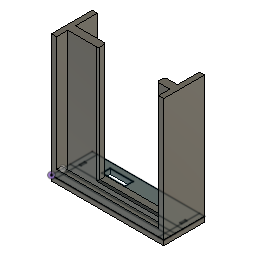
POWERDIAG_OBI_CASE_1 (Autodesk Fusion 360 design; units mm, degrees)
part number: 2026-08-31-19-42-01-999
Autodesk Fusion 360 part; units mm, degrees
sketch "Sketch1" plane through (0, 0, 0) normal (0, 0, 1) x (1, 0, 0)
  line L0 (0, 0) -> (44, 0)
  line L1 (44, 0) -> (44, 16)
  line L2 (44, 16) -> (0, 16)
  line L3 (0, 16) -> (0, 0)
  line L4 (0, 2.6) -> (44, 2.6)
  line L5 (2, 16) -> (2, 0)
  line L6 (42, 16) -> (42, 0)
  line L7 (0, 4.4) -> (44, 4.4)
  line L8 (0, 7.4) -> (44, 7.4)
  line L9 (9.2, 10.6) -> (18.2, 10.6)
  line L10 (18.2, 10.6) -> (18.2, 13.8)
  line L11 (18.2, 13.8) -> (9.2, 13.8)
  line L12 (9.2, 13.8) -> (9.2, 10.6)
  line L13 (2, 11) -> (2.6, 11)
  line L14 (2.6, 11) -> (2.6, 9)
  line L15 (2.6, 9) -> (2, 9)
  line L16 (2, 9) -> (2, 11)
  line L17 (42, 11) -> (41.4, 11)
  line L18 (41.4, 11) -> (41.4, 9)
  line L19 (41.4, 9) -> (42, 9)
  line L20 (42, 9) -> (42, 11)
  dimension "d2" = 16
  dimension "d3" = 2.6
  dimension "d4" = 2
  dimension "d5" = 2
  dimension "d7" = 1.8
  dimension "d8" = 3
  dimension "d9" = 3.2
  dimension "d10" = 3.2
  dimension "d11" = 9
  dimension "d12" = 7.2
  dimension "d13" = 40
  dimension "d22" = 2
  dimension "d23" = 0.6
  dimension "d24" = 1.6
  dimension "d25" = 1.6
  dimension "d26" = 0.6
  dimension "d27" = 2
  constraint horizontal L0
  constraint vertical L1
  constraint horizontal L2
  constraint vertical L3
  constraint coincident L0.start L3.end
  constraint coincident L3 L4.start
  constraint coincident L1 L4.end
  constraint perpendicular L1 L4
  constraint coincident L2 L5.start
  constraint coincident L0 L5.end
  constraint perpendicular L0 L5
  constraint coincident L2 L6.start
  constraint coincident L0 L6.end
  constraint perpendicular L0 L6
  constraint coincident L1 L7.end
  constraint perpendicular L1 L7
  constraint coincident L3 L8.start
  constraint perpendicular L6 L8
  constraint coincident L1 L8.end
  constraint horizontal L9
  constraint vertical L10
  constraint horizontal L11
  constraint vertical L12
  constraint horizontal L13
  constraint vertical L14
  constraint horizontal L15
  constraint vertical L16
  constraint coincident L5 L13.start
  constraint horizontal L17
  constraint vertical L18
  constraint horizontal L19
  constraint vertical L20
  constraint coincident L6 L17.start
  measures "d2" distance of L0.end L1.end
  measures "d3" distance of L0 L4
  measures "d4" distance of L3 L5
  measures "d5" distance of L1 L6
  measures "d7" distance of L4 L7
  measures "d8" distance of L7 L8
  measures "d9" distance of L8 L9
  measures "d10" distance of L9.start L11.end
  measures "d11" distance of L10 L12
  measures "d12" distance of L5 L12
  measures "d13" distance of L5 L6
  measures "d22" distance of L13.end L14.end
  measures "d23" distance of L5 L14
  measures "d24" distance of L8 L15
  measures "d25" distance of L8 L19
  measures "d26" distance of L18 L20
  measures "d27" distance of L17 L19
extrude "Extrude1" add sketch "Sketch1" against normal blind 2
extrude "Extrude2" add sketch "Sketch1" along normal blind 3 contours L0 L3 L4 L5 | L0 L4 L5 L6 | L3 L4 L5 L7 | L0 L1 L4 L6 | L3 L5 L7 L8 | L1 L4 L6 L7 | L5 L6 L7 L8 | L2 L3 L5 L8 L16 | L1 L6 L7 L8 | L1 L2 L6 L8 L20
sketch "Sketch2" plane through (0, 0, 3) normal (0, 0, 1) x (-1, 0, 0)
  line L0 (-2, -4.4) -> (-42, -4.4)
  line L1 (-42, -4.4) -> (-42, -2.6)
  line L2 (-42, -2.6) -> (-2, -2.6)
  line L3 (-2, -2.6) -> (-2, -4.4)
  line L4 (0, -16) -> (0, 0)
  line L5 (0, 0) -> (-44, 0)
  line L6 (-44, 0) -> (-44, -16)
  line L7 (-44, -16) -> (-42, -16)
  line L8 (-42, -16) -> (-42, -7.4)
  line L9 (-42, -7.4) -> (-2, -7.4)
  line L10 (-2, -7.4) -> (-2, -16)
  line L11 (-2, -16) -> (0, -16)
  line L12 (-14, -7.4) -> (-14, -4.4)
  line L13 (-2, -16) -> (-2, 0)
  line L14 (-37, -7.4) -> (-37, -4.4)
  line L15 (-42, -16) -> (-42, 0)
  dimension "d18" = 12
  dimension "d19" = 5
  constraint coincident L9 L12.start
  constraint coincident L0 L12.end
  constraint perpendicular L0 L12
  constraint coincident L9 L14.start
  constraint coincident L0 L14.end
  constraint perpendicular L0 L14
  measures "d18" distance of L12 L13
  measures "d19" distance of L14 L15
extrude "Extrude3" add sketch "Sketch2" along normal blind 45 contours L0 L9 L12 L13 | L3 L4 L5 L10 L11 L13 | L0 L9 L14 L15 | L1 L5 L6 L7 L8 L15
extrude "Extrude4" add sketch "Sketch1" along normal blind 25 contours L5 L13 L14 L15 L16 | L6 L17 L18 L19 L20
chamfer "Chamfer1" distance 0.6 angle 45 8 edges at (2.6, 9, 12.5) (14, 7.4, 25.5) (14, 4.4, 25.5) (41.4, 9, 12.5) (37, 7.4, 25.5) (37, 4.4, 25.5) (22, 2.6, 3) (25.5, 4.4, 3) tangent chain off
